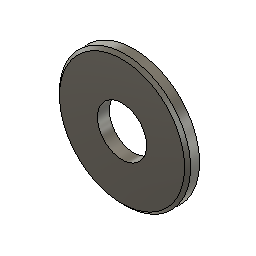
Nudge_1515_High_3mm (Autodesk Fusion 360 archive; units mm, degrees)
design "M3 Fender Washer"
Autodesk Fusion 360 part; units mm, degrees
sketch "Sketch1" plane through (0, 0, 0) normal (0, 0, 1) x (1, 0, 0)
  circle A0 centre (0, 0) radius 4.4
  circle A1 centre (0, 0) radius 1.65
  dimension "d1" = 3.3
  dimension "d2" = 8.8
  constraint coincident A0.centre A1.centre
  constraint concentric A0 A1
  measures "d1" diameter of A1
  measures "d2" diameter of A0
extrude "Extrude1" add sketch "Sketch1" along normal blind 0.8
chamfer "Chamfer1" distance 0.2 angle 45 1 edges at (-4.1022, -1.5911, 0.8) measured on face at (3.4608, -0.3006, 0.8)

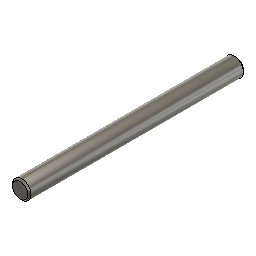
design "m3_pin_main 35mm"
Autodesk Fusion 360 part; units mm, degrees
sketch "Sketch1" plane through (0, 0, 0) normal (0, 0, 1) x (1, 0, 0)
  circle A0 centre (0, 0) radius 1.5
  dimension "d1" = 3
  constraint coincident A0.centre origin
  measures "d1" diameter of A0
extrude "Extrude1" add sketch "Sketch1" along normal blind 35
chamfer "Chamfer1" distance 0.25 angle 45 2 edges at (-1.3985, -0.5424, 35) (-1.3985, -0.5424, 0)

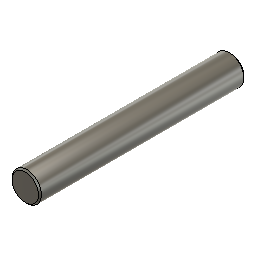
design "M5 Pin 35mm"
Autodesk Fusion 360 part; units mm, degrees
sketch "Sketch1" plane through (0, 0, 0) normal (0, 0, 1) x (1, 0, 0)
  circle A0 centre (0, 0) radius 2.5
  dimension "d1" = 5
  constraint coincident A0.centre origin
  measures "d1" diameter of A0
extrude "Extrude1" add sketch "Sketch1" along normal blind 35
chamfer "Chamfer1" distance 0.25 angle 45 2 edges at (-2.3308, -0.904, 35) (-2.3308, -0.904, 0)

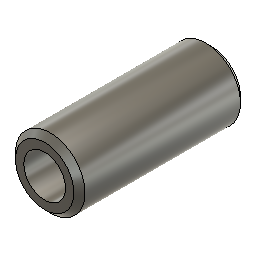
design "Internal-thread 5mm M3 Spacer 12mm long"
Autodesk Fusion 360 part; units mm, degrees
sketch "Sketch1" plane through (0, 0, 0) normal (0, 0, 1) x (1, 0, 0)
  circle A0 centre (0, 0) radius 2.5
  circle A1 centre (0, 0) radius 1.5
  dimension "d1" = 5
  dimension "d2" = 3
  constraint coincident A0.centre A1.centre
  measures "d1" diameter of A0
  measures "d2" diameter of A1
extrude "Extrude1" add sketch "Sketch1" along normal blind 12
extrude "Extrude2" add sketch "Sketch1" along normal blind 2 contours A1
chamfer "Chamfer1" distance 0.4 angle 45 2 edges at (-2.3308, -0.904, 0) (-2.3308, -0.904, 12) measured on face at (2.4969, -0.1246, 8) measured on face at (2.1518, -0.1987, 12)

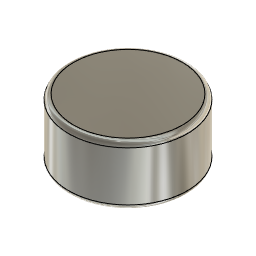
design "6x3mm Magnet"
Autodesk Fusion 360 part; units mm, degrees
sketch "Sketch1" plane through (0, 0, 0) normal (0, 0, 1) x (1, 0, 0)
  circle A0 centre (0, 0) radius 3
  dimension "d1" = 6
  constraint coincident A0.centre origin
  measures "d1" diameter of A0
extrude "Extrude1" add sketch "Sketch1" along normal blind 3
fillet "Fillet1" radius 0.25 2 edges at (-2.797, -1.0848, 3) (-2.797, -1.0848, 0)
